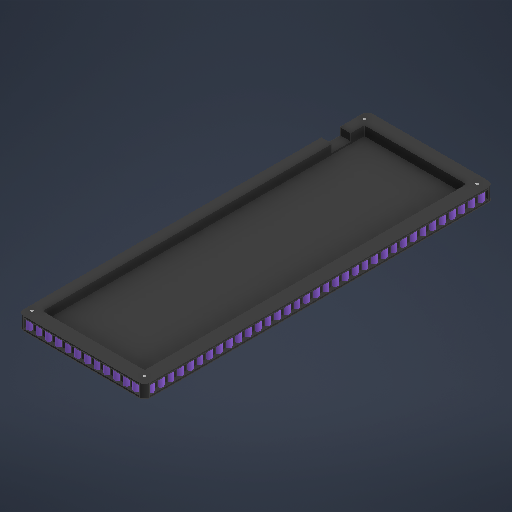
# Autodesk Inventor part: Bottom_Plate_MKey
Saved by Autodesk Inventor 2026 (Build 300175050, 175E)
## iProperties
Created: 2025-06-24
Part Number: Bottom_Plate_MKey
Material: Generic
Document SubType Name: Modeling
Designer: SaiAn
Density: 1 g/cm^3
Appearance: Default
Author: SaiAn
Autodesk Inventor part; units mm, degrees
ref_plane "YZ Plane" through (0, 0, 0) normal (1, 0, 0) x (0, 1, 0)
ref_plane "XZ Plane" through (0, 0, 0) normal (0, 1, 0) x (-1, 0, 0)
ref_plane "XY Plane" through (0, 0, 0) normal (0, 0, 1) x (1, 0, 0)
sketch "Sketch1" plane through (0, 0, 0) normal (0, 1, 0) x (-1, 0, 0)
  line L0 (0, 0) -> (100.47, 0)
  line L1 (100.47, 0) -> (100.47, -315.78)
  line L2 (100.47, -315.78) -> (0, -315.78)
  line L3 (0, -315.78) -> (0, 0)
  line L4 (110.47, 10) -> (-10, 10)
  line L5 (-10, 10) -> (-10, -325.78)
  line L6 (-10, -325.78) -> (110.47, -325.78)
  line L7 (110.47, -325.78) -> (110.47, 10)
  circle A0 centre (105.47, 5) radius 1.7
  circle A1 centre (-5, 5) radius 1.7
  circle A2 centre (-5, -320.78) radius 1.7
  circle A3 centre (105.47, -320.78) radius 1.7
  circle A4 centre (105.47, 5) radius 3
  circle A5 centre (-5, 5) radius 3
  circle A6 centre (-5, -320.78) radius 3
  circle A7 centre (105.47, -320.78) radius 3
  dimension "d0" = 100.47
  dimension "d1" = 315.78
  dimension "d2" = 120.47
  dimension "d3" = 335.78
  dimension "d4" = 10
  dimension "d5" = 10
  dimension "d6" = 3.4
  dimension "d7" = 3.4
  dimension "d8" = 3.4
  dimension "d9" = 3.4
  dimension "d10" = 5
  dimension "d11" = 5
  dimension "d12" = 5
  dimension "d13" = 5
  dimension "d14" = 5
  dimension "d15" = 5
  dimension "d16" = 5
  dimension "d17" = 5
  dimension "d18" = 6
  dimension "d19" = 6
  dimension "d20" = 6
  dimension "d21" = 6
  constraints: 16 end point, 8 centre point, 4 coincident, 4 parallel, 2 horizontal, 2 perpendicular
  measures "d0" distance of L1.end L2.end
  measures "d1" distance of L0.end L1.end
  measures "d2" distance of L6.end L5.end
  measures "d3" distance of L5.end L4.end
  measures "d4" distance between parallel lines of L1 L7
  measures "d5" distance between parallel lines of L6 L2
  measures "d6" diameter of A0
  measures "d7" diameter of A1
  measures "d8" diameter of A2
  measures "d9" diameter of A3
  measures "d10" distance from line of L7 A0.centre
  measures "d11" distance from line of L4 A0.centre
  measures "d12" distance from line of L5 A1.centre
  measures "d13" distance from line of L4 A1.centre
  measures "d14" distance from line of L5 A2.centre
  measures "d15" distance from line of L6 A2.centre
  measures "d16" distance from line of L7 A3.centre
  measures "d17" distance from line of L6 A3.centre
  measures "d18" diameter of A4
  measures "d19" diameter of A5
  measures "d20" diameter of A6
  measures "d21" diameter of A7
extrude "Extrusion1" add sketch "Sketch1" along normal blind 13 contours A4 | A5 | A6 | A7
extrude "Extrusion2" cut sketch "Sketch1" along normal blind 3.1 contours A4 | A5 | A6 | A7
extrude "Extrusion3" add sketch "Sketch1" along normal blind 13 contours L7 L6 L5 L4
extrude "Extrusion4" add sketch "Sketch1" along normal blind 3 contours L0 L1 L2 L3
sketch "Sketch3" plane through (0, 13, 0) normal (0, 1, 0) x (1, 0, 0)
  line L0 (-100.47, 0) -> (-100.47, 315.78) projected
  line L1 (-110.47, 325.78) -> (-110.47, -10) projected
  line L2 (-100.47, 302.18) -> (-110.47, 302.18)
  line L3 (-110.47, 302.18) -> (-110.47, 283.68)
  line L4 (-110.47, 283.68) -> (-100.47, 283.68)
  line L5 (-100.47, 283.68) -> (-100.47, 302.18)
  line L6 (10, 325.78) -> (-110.47, 325.78) projected
  point P0 (0, 0)
  dimension "d30" = 18.5
  dimension "d31" = 23.6
  constraints: 8 end point, 2 parallel, 2 point on line, 1 horizontal, 1 perpendicular
  measures "d30" distance of L3.end L2.end
  measures "d31" distance between parallel lines of L6 L2
extrude "Extrusion5" cut sketch "Sketch3" against normal blind 7.5
sketch "Sketch7" plane through (-110.47, 0, 10) normal (0, 0, 1) x (1, 0, 0)
  line L0 (0, 0) -> (0, 13) projected
  line L1 (120.47, 0) -> (120.47, 13) projected
  line L2 (0, 13) -> (120.47, 13)
  line L3 (120.47, 13) -> (120.47, 0)
  line L4 (120.47, 0) -> (0, 0)
  line L5 (0, 0) -> (0, 13)
  point P0 (110.47, 0)
  constraints: 8 end point, 2 parallel, 1 horizontal, 1 perpendicular
extrude "Extrusion7" add sketch "Sketch7" along normal blind 3
sketch "Sketch8" plane through (10, 0, -325.78) normal (1, 0, 0) x (0, 0, -1)
  line L0 (0, 13) -> (-338.78, 13) projected
  line L1 (0, 0) -> (0, 13) projected
  line L2 (-338.78, 13) -> (0, 13)
  line L3 (0, 13) -> (0, 0)
  line L4 (0, 0) -> (-338.78, 0)
  line L5 (-338.78, 0) -> (-338.78, 13)
  point P0 (-325.78, 0)
  constraints: 8 end point, 2 parallel, 1 horizontal, 1 perpendicular
extrude "Extrusion8" add sketch "Sketch8" along normal blind 3
sketch "Sketch9" plane through (-110.47, 0, -325.78) normal (0, 0, -1) x (-1, 0, 0)
  line L0 (0, 13) -> (-123.47, 13) projected
  line L1 (-123.47, 13) -> (0, 13)
  line L2 (0, 13) -> (0, 0)
  line L3 (0, 0) -> (-123.47, 0)
  line L4 (-123.47, 0) -> (-123.47, 13)
  point P0 (-110.47, 0)
  constraints: 8 end point, 2 parallel, 1 horizontal, 1 perpendicular
extrude "Extrusion9" add sketch "Sketch9" along normal blind 3
fillet "Fillet3" radius 5 4 edges at (13, 6.5, 13) (-110.47, 6.5, 13) (13, 6.5, -328.78) (-110.47, 6.5, -328.78)
sketch "Sketch10" plane through (-110.47, 0, 13) normal (0, 0, 1) x (1, 0, 0)
  line L0 (5, 0) -> (5, 13) projected
  line L1 (118.47, 13) -> (118.47, 0) projected
  line L2 (5, 2) -> (118.47, 2)
  line L3 (118.47, 2) -> (118.47, 11)
  line L4 (118.47, 11) -> (5, 11)
  line L5 (5, 11) -> (5, 2)
  point P0 (110.47, 0)
  dimension "d56" = 9
  constraints: 8 end point, 2 parallel, 2 point on line, 1 horizontal, 1 perpendicular
  measures "d56" distance of L3.end L2.end
extrude "Extrusion10" cut sketch "Sketch10" against normal blind 3
sketch "Sketch11" plane through (13, 0, -325.78) normal (1, 0, 0) x (0, 0, -1)
  line L0 (-333.78, 13) -> (-333.78, 0) projected
  line L1 (-2, 0) -> (-2, 13) projected
  line L2 (-333.78, 2) -> (-2, 2)
  line L3 (-2, 2) -> (-2, 11)
  line L4 (-2, 11) -> (-333.78, 11)
  line L5 (-333.78, 11) -> (-333.78, 2)
  point P0 (-325.78, 0)
  dimension "d59" = 9
  constraints: 8 end point, 2 parallel, 2 point on line, 1 horizontal, 1 perpendicular
  measures "d59" distance of L3.end L2.end
extrude "Extrusion11" cut sketch "Sketch11" against normal blind 3
sketch "Sketch12" plane through (-110.47, 0, -328.78) normal (0, 0, -1) x (-1, 0, 0)
  line L0 (-118.47, 0) -> (-118.47, 13) projected
  line L1 (-5, 13) -> (-5, 0) projected
  line L2 (-118.47, 2) -> (-5, 2)
  line L3 (-5, 2) -> (-5, 11)
  line L4 (-5, 11) -> (-118.47, 11)
  line L5 (-118.47, 11) -> (-118.47, 2)
  point P0 (-110.47, 0)
  dimension "d62" = 9
  constraints: 8 end point, 2 parallel, 2 point on line, 1 horizontal, 1 perpendicular
  measures "d62" distance of L3.end L2.end
extrude "Extrusion12" cut sketch "Sketch12" against normal blind 3
sketch "Sketch13" plane through (-105.47, 2, 13) normal (0, 1, 0) x (1, 0, 0)
  line L0 (113.47, 3) -> (0, 3) projected
  circle A0 centre (3.2242, 3) radius 3
  line L1 (113.47, 0) -> (0, 0) projected
  circle A1 centre (12.7242, 3) radius 3
  circle A2 centre (22.2242, 3) radius 3
  circle A3 centre (31.7242, 3) radius 3
  circle A4 centre (41.2242, 3) radius 3
  circle A5 centre (50.7242, 3) radius 3
  circle A6 centre (60.2242, 3) radius 3
  circle A7 centre (69.7242, 3) radius 3
  circle A8 centre (79.2242, 3) radius 3
  circle A9 centre (88.7242, 3) radius 3
  circle A10 centre (98.2242, 3) radius 3
  circle A11 centre (107.7242, 3) radius 3
  line L2 (0.2242, 3) -> (110.7242, 3)
  point P0 (105.47, 13)
  point P1 (104.7242, 3)
  point P2 (101.2242, 3)
  point P3 (95.2242, 3)
  point P4 (91.7242, 3)
  point P5 (85.7242, 3)
  point P6 (82.2242, 3)
  point P7 (76.2242, 3)
  point P8 (72.7242, 3)
  point P9 (66.7242, 3)
  point P10 (63.2242, 3)
  point P11 (57.2242, 3)
  point P12 (53.7242, 3)
  point P13 (47.7242, 3)
  point P14 (44.2242, 3)
  point P15 (38.2242, 3)
  point P16 (34.7242, 3)
  point P17 (28.7242, 3)
  point P18 (25.2242, 3)
  point P19 (19.2242, 3)
  point P20 (15.7242, 3)
  point P21 (9.7242, 3)
  point P22 (6.2242, 3)
  dimension "d67" = 9.5
  constraints: 10 centre point, 2 end point, 2 horizontal, 2 tangent, 30 other
  measures "d67" distance of point (3.224, 3) A1.centre
extrude "Extrusion13" add sketch "Sketch13" along normal blind 9 contours A0 L0 | L0 A1 | L0 A2 | A3 L0 | A4 L0 | A5 L0 | A6 L0 | A7 L0 | A8 L0 | A9 L0 | A10 L0 | A11 L0 picked at (2.4424, 2.3765) picked at (12.5017, 2.0251) picked at (22.4467, 2.0251) picked at (30.9424, 1.9315) picked at (42.2242, 1.753) picked at (51.6502, 2.3436) picked at (61.1502, 2.3436) picked at (68.7982, 2.3436) picked at (78.2982, 2.3436) picked at (87.7982, 2.3436) picked at (97.2982, 2.3436) picked at (106.7982, 2.3436)
sketch "Sketch14" plane through (13, 2, 8) normal (0, 1, 0) x (1, 0, 0)
  circle A0 centre (-2.9902, 4.0486) radius 2.9902
  line L0 (0, 331.78) -> (0, 0) projected
  circle A1 centre (-2.9902, 13.5486) radius 2.9902
  circle A2 centre (-2.9902, 23.0486) radius 2.9902
  circle A3 centre (-2.9902, 32.5486) radius 2.9902
  circle A4 centre (-2.9902, 42.0486) radius 2.9902
  circle A5 centre (-2.9902, 51.5486) radius 2.9902
  circle A6 centre (-2.9902, 61.0486) radius 2.9902
  circle A7 centre (-2.9902, 70.5486) radius 2.9902
  circle A8 centre (-2.9902, 80.0486) radius 2.9902
  circle A9 centre (-2.9902, 89.5486) radius 2.9902
  circle A10 centre (-2.9902, 99.0486) radius 2.9902
  circle A11 centre (-2.9902, 108.5486) radius 2.9902
  circle A12 centre (-2.9902, 118.0486) radius 2.9902
  circle A13 centre (-2.9902, 127.5486) radius 2.9902
  circle A14 centre (-2.9902, 137.0486) radius 2.9902
  circle A15 centre (-2.9902, 146.5486) radius 2.9902
  circle A16 centre (-2.9902, 156.0486) radius 2.9902
  circle A17 centre (-2.9902, 165.5486) radius 2.9902
  circle A18 centre (-2.9902, 175.0486) radius 2.9902
  circle A19 centre (-2.9902, 184.5486) radius 2.9902
  circle A20 centre (-2.9902, 194.0486) radius 2.9902
  circle A21 centre (-2.9902, 203.5486) radius 2.9902
  circle A22 centre (-2.9902, 213.0486) radius 2.9902
  circle A23 centre (-2.9902, 222.5486) radius 2.9902
  circle A24 centre (-2.9902, 232.0486) radius 2.9902
  circle A25 centre (-2.9902, 241.5486) radius 2.9902
  circle A26 centre (-2.9902, 251.0486) radius 2.9902
  circle A27 centre (-2.9902, 260.5486) radius 2.9902
  circle A28 centre (-2.9902, 270.0486) radius 2.9902
  circle A29 centre (-2.9902, 279.5486) radius 2.9902
  circle A30 centre (-2.9902, 289.0486) radius 2.9902
  circle A31 centre (-2.9902, 298.5486) radius 2.9902
  circle A32 centre (-2.9902, 308.0486) radius 2.9902
  circle A33 centre (-2.9902, 317.5486) radius 2.9902
  circle A34 centre (-2.9902, 327.0486) radius 2.9902
  line L1 (-3, 331.78) -> (-3, 0) projected
  line L2 (-3, 1.0584) -> (-3, 330.0389)
  point P0 (-13, 8)
  point P1 (-3, 324.0584)
  point P2 (-3, 320.5389)
  point P3 (-3, 314.5584)
  point P4 (-3, 311.0389)
  point P5 (-3, 305.0584)
  point P6 (-3, 301.5389)
  point P7 (-3, 295.5584)
  point P8 (-3, 292.0389)
  point P9 (-3, 286.0584)
  point P10 (-3, 282.5389)
  point P11 (-3, 276.5584)
  point P12 (-3, 273.0389)
  point P13 (-3, 267.0584)
  point P14 (-3, 263.5389)
  point P15 (-3, 257.5584)
  point P16 (-3, 254.0389)
  point P17 (-3, 248.0584)
  point P18 (-3, 244.5389)
  point P19 (-3, 238.5584)
  point P20 (-3, 235.0389)
  point P21 (-3, 229.0584)
  point P22 (-3, 225.5389)
  point P23 (-3, 219.5584)
  point P24 (-3, 216.0389)
  point P25 (-3, 210.0584)
  point P26 (-3, 206.5389)
  point P27 (-3, 200.5584)
  point P28 (-3, 197.0389)
  point P29 (-3, 191.0584)
  point P30 (-3, 187.5389)
  point P31 (-3, 181.5584)
  point P32 (-3, 178.0389)
  point P33 (-3, 172.0584)
  point P34 (-3, 168.5389)
  point P35 (-3, 162.5584)
  point P36 (-3, 159.0389)
  point P37 (-3, 153.0584)
  point P38 (-3, 149.5389)
  point P39 (-3, 143.5584)
  point P40 (-3, 140.0389)
  point P41 (-3, 134.0584)
  point P42 (-3, 130.5389)
  point P43 (-3, 124.5584)
  point P44 (-3, 121.0389)
  point P45 (-3, 115.0584)
  point P46 (-3, 111.5389)
  point P47 (-3, 105.5584)
  point P48 (-3, 102.0389)
  point P49 (-3, 96.0584)
  point P50 (-3, 92.5389)
  point P51 (-3, 86.5584)
  point P52 (-3, 83.0389)
  point P53 (-3, 77.0584)
  point P54 (-3, 73.5389)
  point P55 (-3, 67.5584)
  point P56 (-3, 64.0389)
  point P57 (-3, 58.0584)
  point P58 (-3, 54.5389)
  point P59 (-3, 48.5584)
  point P60 (-3, 45.0389)
  point P61 (-3, 39.0584)
  point P62 (-3, 35.5389)
  point P63 (-3, 29.5584)
  point P64 (-3, 26.0389)
  point P65 (-3, 20.0584)
  point P66 (-3, 16.5389)
  point P67 (-3, 10.5584)
  point P68 (-3, 7.0389)
  dimension "d76" = 9.5
  constraints: 33 centre point, 2 end point, 2 tangent, 2 vertical, 74 other
  measures "d76" distance of point (-2.99, 4.049) A1.centre
extrude "Extrusion14" add sketch "Sketch14" along normal blind 9 contours L1 A0 | A1 L1 | A2 L1 | A3 L1 | A4 L1 | A5 L1 | A6 L1 | A7 L1 | A8 L1 | A9 L1 | A10 L1 | A11 L1 | A12 L1 | A13 L1 | A14 L1 | A15 L1 | A16 L1 | A17 L1 | A18 L1 | A19 L1 | A20 L1 | A21 L1 | A22 L1 | A23 L1 | A24 L1 | A25 L1 | A26 L1 | A27 L1 | A28 L1 | A29 L1 | A30 L1 | A31 L1 | A32 L1 | A33 L1 | A34 L1 picked at (-1.7737, 4.6711) picked at (-2.1544, 14.3534) picked at (-1.8028, 23.2952) picked at (-1.8028, 32.7952) picked at (-1.996, 41.4504) picked at (-1.996, 50.9504) picked at (-1.996, 60.4504) picked at (-1.9321, 71.329) picked at (-1.9321, 80.829) picked at (-1.9321, 90.329) picked at (-1.9321, 99.829) picked at (-1.9321, 109.329) picked at (-1.9321, 118.829) picked at (-1.7208, 126.6948) picked at (-1.7777, 137.0242) picked at (-1.7777, 146.5242) picked at (-1.7777, 156.0242) picked at (-1.7777, 165.5242) picked at (-1.7777, 175.0242) picked at (-1.7777, 184.5242) picked at (-1.7777, 194.0242) picked at (-1.7777, 203.5242) picked at (-1.7777, 213.0242) picked at (-1.7777, 222.5242) picked at (-1.7777, 232.0242) picked at (-1.7777, 241.5242) picked at (-1.7777, 251.0242) picked at (-2.5664, 261.4476) picked at (-2.5664, 270.9476) picked at (-2.5664, 280.4476) picked at (-2.5664, 289.9476) picked at (-2.5664, 299.4476) picked at (-2.5664, 308.9476) picked at (-2.5664, 318.4476) picked at (-1.7777, 327.0242)
sketch "Sketch15" plane through (-105.47, 2, -328.78) normal (0, 1, 0) x (1, 0, 0)
  circle A0 centre (109.4627, -2.9451) radius 2.9451
  line L0 (0, 0) -> (113.47, 0) projected
  circle A1 centre (99.9627, -2.9451) radius 2.9451
  circle A2 centre (90.4627, -2.9451) radius 2.9451
  circle A3 centre (80.9627, -2.9451) radius 2.9451
  circle A4 centre (71.4627, -2.9451) radius 2.9451
  circle A5 centre (61.9627, -2.9451) radius 2.9451
  circle A6 centre (52.4627, -2.9451) radius 2.9451
  circle A7 centre (42.9627, -2.9451) radius 2.9451
  circle A8 centre (33.4627, -2.9451) radius 2.9451
  circle A9 centre (23.9627, -2.9451) radius 2.9451
  circle A10 centre (14.4627, -2.9451) radius 2.9451
  circle A11 centre (4.9627, -2.9451) radius 2.9451
  line L1 (0, -3) -> (113.47, -3) projected
  line L2 (112.4073, -3) -> (2.0181, -3)
  point P0 (105.47, -328.78)
  point P1 (7.9073, -3)
  point P2 (11.5181, -3)
  point P3 (17.4073, -3)
  point P4 (21.0181, -3)
  point P5 (26.9073, -3)
  point P6 (30.5181, -3)
  point P7 (36.4073, -3)
  point P8 (40.0181, -3)
  point P9 (45.9073, -3)
  point P10 (49.5181, -3)
  point P11 (55.4073, -3)
  point P12 (59.0181, -3)
  point P13 (64.9073, -3)
  point P14 (68.5181, -3)
  point P15 (74.4073, -3)
  point P16 (78.0181, -3)
  point P17 (83.9073, -3)
  point P18 (87.5181, -3)
  point P19 (93.4073, -3)
  point P20 (97.0181, -3)
  point P21 (102.9073, -3)
  point P22 (106.5181, -3)
  dimension "d85" = 9.5
  constraints: 10 centre point, 2 end point, 2 horizontal, 2 tangent, 29 other
  measures "d85" distance of point (109.463, -2.945) A1.centre
extrude "Extrusion15" add sketch "Sketch15" along normal blind 9 contours L1 A0 | L1 A1 | A2 L1 | A3 L1 | A4 L1 | A5 L1 | A6 L1 | A7 L1 | A8 L1 | A9 L1 | A10 L1 | A11 L1 picked at (108.6643, -2.1411) picked at (100.9133, -1.5107) picked at (91.4133, -1.5107) picked at (81.9133, -1.5107) picked at (72.4133, -1.5107) picked at (62.6418, -1.545) picked at (53.4386, -2.1233) picked at (43.9386, -2.1233) picked at (34.3683, -2.3343) picked at (24.5749, -2.2081) picked at (15.2303, -2.3635) picked at (5.5748, -2.2142)
sketch "Sketch17" plane through (0, 0, 0) normal (0, -1, 0) x (1, 0, 0)
  line L0 (-0.493, -49.5364) -> (-0.493, -2478.3068) construction
  line L1 (-0.493, -2478.3068) -> (-8355.222, -2478.3068) construction
  line L2 (-8355.222, -2478.3068) -> (-8355.222, -49.5364) construction
  line L3 (-8355.222, -49.5364) -> (-0.493, -49.5364) construction
  line L4 (-86.4104, -117.6297) -> (-86.4104, -104.5401)
  line L5 (-86.4104, -104.5401) -> (-52.1548, -83.6526)
  line L6 (-52.1548, -83.6526) -> (-86.4104, -62.3474)
  line L7 (-86.4104, -62.3474) -> (-86.4104, -50.0237)
  line L8 (-86.4104, -50.0237) -> (-43.3821, -77.3864)
  line L9 (-43.3821, -77.3864) -> (-0.493, -50.8592)
  line L10 (-0.493, -50.8592) -> (-0.493, -63.9487)
  line L11 (-0.493, -63.9487) -> (-34.1219, -84.4185)
  line L12 (-34.1219, -84.4185) -> (-0.493, -105.306)
  line L13 (-0.493, -105.306) -> (-0.493, -117.6297)
  line L14 (-0.493, -117.6297) -> (-42.8251, -90.7544)
  line L15 (-42.8251, -90.7544) -> (-86.4104, -117.6297)
  line L16 (-86.4104, -186.2103) -> (-86.4104, -173.1208)
  line L17 (-86.4104, -173.1208) -> (-52.1548, -152.2333)
  line L18 (-52.1548, -152.2333) -> (-86.4104, -130.928)
  line L19 (-86.4104, -130.928) -> (-86.4104, -118.6044)
  line L20 (-86.4104, -118.6044) -> (-43.3821, -145.9671)
  line L21 (-43.3821, -145.9671) -> (-0.493, -119.4399)
  line L22 (-0.493, -119.4399) -> (-0.493, -132.5294)
  line L23 (-0.493, -132.5294) -> (-34.1219, -152.9992)
  line L24 (-34.1219, -152.9992) -> (-0.493, -173.8867)
  line L25 (-0.493, -173.8867) -> (-0.493, -186.2103)
  line L26 (-0.493, -186.2103) -> (-42.8251, -159.3351)
  line L27 (-42.8251, -159.3351) -> (-86.4104, -186.2103)
  line L28 (-86.4104, -254.791) -> (-86.4104, -241.7015)
  line L29 (-86.4104, -241.7015) -> (-52.1548, -220.814)
  line L30 (-52.1548, -220.814) -> (-86.4104, -199.5087)
  line L31 (-86.4104, -199.5087) -> (-86.4104, -187.1851)
  line L32 (-86.4104, -187.1851) -> (-43.3821, -214.5477)
  line L33 (-43.3821, -214.5477) -> (-0.493, -188.0206)
  line L34 (-0.493, -188.0206) -> (-0.493, -201.1101)
  line L35 (-0.493, -201.1101) -> (-34.1219, -221.5799)
  line L36 (-34.1219, -221.5799) -> (-0.493, -242.4674)
  line L37 (-0.493, -242.4674) -> (-0.493, -254.791)
  line L38 (-0.493, -254.791) -> (-42.8251, -227.9158)
  line L39 (-42.8251, -227.9158) -> (-86.4104, -254.791)
  point P0 (0, 0)
  dimension "d0" = 100.47
  dimension "d1" = 315.78
  dimension "d2" = 120.47
  dimension "d3" = 335.78
  dimension "d4" = 10
  dimension "d5" = 10
  dimension "d6" = 3.4
  dimension "d7" = 3.4
  dimension "d8" = 3.4
  dimension "d9" = 3.4
  dimension "d10" = 5
  dimension "d11" = 5
  dimension "d12" = 5
  dimension "d13" = 5
  dimension "d14" = 5
  dimension "d15" = 5
  dimension "d16" = 5
  dimension "d17" = 5
  dimension "d18" = 6
  dimension "d19" = 6
  dimension "d20" = 6
  dimension "d21" = 6
  constraints: 2 other
extrude "Extrusion16" cut sketch "Sketch17" against normal blind 0.2
body "Solid1"
